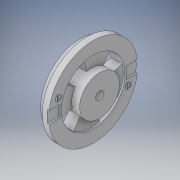
# Autodesk Inventor part: Motor Endcap
Saved by Autodesk Inventor 2016 (Build 200138000, 138)
## iProperties
Created: 2015-05-20
Part Number: Motor Endcap
Material: Generic
Document SubType Name: Modeling
Designer: jonathan
Density: 1 g/cm^3
Appearance: PTFE
Author: jonathan
Autodesk Inventor part; units mm, degrees
ref_plane "XZ Plane" through (0, 0, 0) normal (0, 1, 0) x (-1, 0, 0)
ref_plane "XY Plane" through (0, 0, 0) normal (0, 0, 1) x (1, 0, 0)
sketch "Sketch1" plane through (0, 0, 0) normal (1, 0, 0) x (0, 1, 0)
  circle A0 centre (0, 0) radius 17.78
  dimension "d0" = 35.56
  constraints: 1 centre point, 1 coincident
  measures "d0" diameter of A0
extrude "Extrusion1" add sketch "Sketch1" along normal blind 2.54
sketch "Sketch2" plane through (0, 0, 0) normal (1, 0, 0) x (0, 1, 0)
  circle A0 centre (0, 0) radius 16.51
  dimension "d3" = 33.02
  constraints: 1 centre point, 1 coincident
  measures "d3" diameter of A0
ref_plane "Work Plane1" through (-2.54, 0, 0) normal (1, 0, 0) x (0, 1, 0)
sketch "Sketch3" plane through (-2.54, 0, 0) normal (1, 0, 0) x (0, 1, 0)
  circle A0 centre (0, 0) radius 15.875
  dimension "d5" = 31.75
  constraints: 1 centre point, 1 coincident
  measures "d5" diameter of A0
loft "Loft1" add profiles "Sketch2", "Sketch3"
sketch "Sketch4" plane through (2.54, 0, 0) normal (1, 0, 0) x (0, 0, -1)
  circle A0 centre (0, 0) radius 7.9375
  dimension "d10" = 15.875
  constraints: 1 centre point, 1 coincident
  measures "d10" diameter of A0
extrude "Extrusion2" add sketch "Sketch4" along normal blind 2.54
sketch "Sketch5" plane through (5.08, 0, 0) normal (1, 0, 0) x (0, 0, -1)
  circle A0 centre (0, 0) radius 7.9375
  circle A1 centre (0, 0) radius 12.7
  line L0 (17.78, -2.3813) -> (17.78, 2.3813)
  line L1 (-17.78, 2.3812) -> (-17.78, -2.3813)
  circle A2 centre (0, 0) radius 17.78 projected
  line L2 (17.78, 2.3813) -> (13.1207, 2.3813)
  line L3 (-13.1207, 2.3812) -> (-17.78, 2.3812)
  line L4 (-17.78, -2.3813) -> (-13.1207, -2.3813)
  line L5 (13.1207, -2.3813) -> (17.78, -2.3813)
  arc A3 (-13.1207, 2.3812) -> (-13.1207, -2.3813) centre (0, 0) ccw
  arc A4 (13.1207, -2.3813) -> (13.1207, 2.3813) centre (0, 0) ccw
  dimension "d13" = 25.4
  dimension "d14" = 15.875
  constraints: 12 end point, 5 parallel, 4 centre point, 4 point on circle, 3 coincident, 2 horizontal, 2 perpendicular, 2 tangent
  measures "d13" diameter of A1
  measures "d14" diameter of A0
extrude "Extrusion3" cut sketch "Sketch5" against normal blind 3.175 contours A1
extrude "Extrusion4" cut sketch "Sketch5" against normal blind 3.175 contours L5 A2 L0 | A2 L2 L0 | A2 L5 A4 L2 | L4 L1 A2 | A2 L3 A3 L4 | A2 L1 L3
sketch "Sketch7" plane through (2.54, 0, 0) normal (1, 0, 0) x (0, 0, -1)
  line L0 (-13.7354, 6.0289) -> (-13.7354, 3.5402)
  line L1 (-14.2434, 3.5402) -> (-14.2434, 6.0289)
  arc A0 (-13.7354, 3.5402) -> (-13.7354, 6.0289) centre (-13.9894, 4.7845) ccw
  arc A1 (-14.2434, 6.0289) -> (-14.2434, 3.5402) centre (-13.9894, 4.7845) ccw
  line L2 (12.7703, -5.0327) -> (13.7606, -5.0327)
  line L3 (14.2686, -5.0327) -> (15.259, -5.0327)
  line L4 (15.259, -4.5247) -> (14.2686, -4.5247)
  line L5 (13.7606, -4.5247) -> (12.7703, -4.5247)
  arc A2 (12.7703, -5.0327) -> (13.7606, -6.0231) centre (14.0146, -4.7787) ccw
  arc A3 (14.2686, -6.0231) -> (15.259, -5.0327) centre (14.0146, -4.7787) ccw
  line L6 (14.2686, -6.0231) -> (14.2686, -5.0327)
  line L7 (14.2686, -4.5247) -> (14.2686, -3.5344)
  line L8 (13.7606, -3.5344) -> (13.7606, -4.5247)
  line L9 (13.7606, -5.0327) -> (13.7606, -6.0231)
  arc A4 (15.259, -4.5247) -> (14.2686, -3.5344) centre (14.0146, -4.7787) ccw
  arc A5 (13.7606, -3.5344) -> (12.7703, -4.5247) centre (14.0146, -4.7787) ccw
  point P0 (0, 0)
  dimension "d24" = 0.254
  dimension "d25" = 0.254
  constraints: 20 end point, 12 point on circle, 9 parallel, 6 centre point, 2 horizontal
  measures "d24" distance from line of L1 A0.centre
  measures "d25" distance from line of L0 A0.centre
extrude "Extrusion5" cut sketch "Sketch7" against normal blind 0.127
sketch "Sketch8" plane through (5.08, 0, 0) normal (1, 0, 0) x (0, 0, -1)
  circle A0 centre (0, 0) radius 1.5875
  arc A1 (-2.0163, 7.6771) -> (-6.4794, 4.585) centre (0, 0) ccw
  arc A2 (-3.2261, 12.2834) -> (-10.367, 7.3359) centre (0, 0) ccw
  circle A3 centre (0, 0) radius 12.7 projected
  line L0 (-2.0163, 7.6771) -> (-3.2261, 12.2834)
  line L1 (-6.4794, 4.585) -> (-10.367, 7.3359)
  dimension "d32" = 3.175
  dimension "d34" = 15.875
  constraints: 6 point on circle, 4 end point, 3 centre point, 3 coincident
  measures "d32" diameter of A0
  measures "d34" diameter of A1
extrude "Extrusion6" cut sketch "Sketch8" against normal through all contours A0 | A1 L1 A2 L0
pattern_circular "Circular Pattern1" count 4 over 360 about axis through (2.54, 0, 0) along (1, 0, 0) of "Extrusion6"
body "Solid1"
